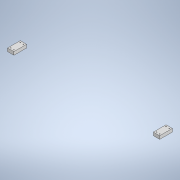
# Autodesk Inventor part: Intake - Lexan Raiser
Saved by Autodesk Inventor 2020 (Build 240168000, 168)
## iProperties
Created: 2020-02-04
Part Number: Intake - Lexan Raiser
Material: Generic
Document SubType Name: Modeling
Designer: aidan
Density: 1 g/cm^3
Appearance: Default
Author: aidan
Autodesk Inventor part; units mm, degrees
ref_plane "YZ Plane" through (0, 0, 0) normal (1, 0, 0) x (0, 1, 0)
ref_plane "XZ Plane" through (0, 0, 0) normal (0, 1, 0) x (-1, 0, 0)
sketch "Sketch2" plane through (0, 0, 0) normal (0, 1, 0) x (-1, 0, 0)
  line L0 (0, 0) -> (-25.4, 0)
  line L1 (-25.4, 0) -> (-25.4, -50.8)
  line L2 (-25.4, -50.8) -> (0, -50.8)
  line L3 (0, -50.8) -> (0, 0)
  dimension "d0" = 50.8
  dimension "d4" = 25.4
  constraints: 8 end point, 2 parallel, 1 horizontal, 1 perpendicular
  measures "d0" distance between parallel lines of L0 L2
  measures "d4" distance between parallel lines of L1 L3
extrude "Extrusion1" add sketch "Sketch2" along normal blind 12.7
sketch "Sketch4" plane through (0, 12.7, 0) normal (0, 1, 0) x (1, 0, 0)
  line L0 (6.35, 6.35) -> (19.05, 6.35) construction
  line L1 (19.05, 6.35) -> (19.05, 44.45) construction
  line L2 (19.05, 44.45) -> (6.35, 44.45) construction
  line L3 (6.35, 44.45) -> (6.35, 6.35) construction
  line L4 (0, 50.8) -> (0, 0) construction
  line L5 (25.4, 50.8) -> (0, 50.8) construction
  line L6 (0, 0) -> (25.4, 0) construction
  line L7 (25.4, 0) -> (25.4, 50.8) construction
  dimension "d5" = 6.35
  dimension "d6" = 6.35
  dimension "d7" = 6.35
  dimension "d8" = 6.35
  constraints: 8 end point, 2 parallel, 1 horizontal, 1 perpendicular
  measures "d5" distance between parallel lines of L4 L3
  measures "d6" distance between parallel lines of L5 L2
  measures "d7" distance between parallel lines of L6 L0
  measures "d8" distance between parallel lines of L7 L1
hole "Hole1" at (6.35, 12.7, -6.35) at (19.05, 12.7, -6.35) at (19.05, 12.7, -44.45) at (6.35, 12.7, -44.45) direction (0, -1, 0) diameter 3.175 end through all
ref_plane "Work Plane1" through (-279.4, 0, -50.8) normal (-1, 0, 0) x (0, 0, 1)
mirror "Mirror1" about plane through (-279.4, 0, -50.8) normal (-1, 0, 0)
body "Solid1"
